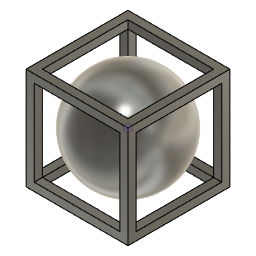
boxspherical (Autodesk Fusion 360 design; units mm, degrees)
Autodesk Fusion 360 part; units mm, degrees
sketch "Sketch1" plane through (0, 0, 0) normal (0, 1, 0) x (1, 0, 0)
  line L0 (12.5, -12.5) -> (-12.5, -12.5)
  line L1 (-12.5, -12.5) -> (-12.5, 12.5)
  line L2 (-12.5, 12.5) -> (12.5, 12.5)
  line L3 (12.5, 12.5) -> (12.5, -12.5)
  line L4 (12.5, -12.5) -> (-12.5, 12.5) construction
  line L5 (-12.5, -12.5) -> (12.5, 12.5) construction
  dimension "d1" = 25
  dimension "d2" = 25
  constraint horizontal L0
  constraint perpendicular L0 L1
  constraint parallel L0 L2
  constraint parallel L1 L3
  constraint coincident L4 origin
  constraint coincident L5 origin
  measures "d1" distance of L0.end L1.end
  measures "d2" distance of L1.end L2.end
extrude "Extrude1" add sketch "Sketch1" along normal mid plane 25 makes body 1
sketch "Sketch2" plane through (0, -12.5, 0) normal (0, -1, 0) x (1, 0, 0)
  line L0 (-12.5, -12.5) -> (12.5, -12.5)
  line L1 (12.5, -12.5) -> (12.5, 12.5)
  line L2 (12.5, 12.5) -> (-12.5, 12.5)
  line L3 (-12.5, 12.5) -> (-12.5, -12.5)
  line L4 (-10.5, -10.5) -> (10.5, -10.5)
  line L5 (10.5, -10.5) -> (10.5, 10.5)
  line L6 (10.5, 10.5) -> (-10.5, 10.5)
  line L7 (-10.5, 10.5) -> (-10.5, -10.5)
  dimension "d6" = -2
extrude "Extrude2" cut sketch "Sketch2" against normal blind 45 contours L4 L5 L6 L7 bodies 1
sketch "Sketch3" plane through (0, 0, 12.5) normal (0, 0, 1) x (-1, 0, 0)
  line L0 (12.5, 12.5) -> (-12.5, 12.5)
  line L1 (-12.5, 12.5) -> (-12.5, -12.5)
  line L2 (-12.5, -12.5) -> (12.5, -12.5)
  line L3 (12.5, -12.5) -> (12.5, 12.5)
  line L4 (10.5, 10.5) -> (-10.5, 10.5)
  line L5 (-10.5, 10.5) -> (-10.5, -10.5)
  line L6 (-10.5, -10.5) -> (10.5, -10.5)
  line L7 (10.5, -10.5) -> (10.5, 10.5)
  dimension "d9" = -2
extrude "Extrude3" cut sketch "Sketch3" against normal blind 41 contours L4 L5 L6 L7 bodies 1
sketch "Sketch4" plane through (12.5, 0, 0) normal (1, 0, 0) x (0, 1, 0)
  line L0 (-12.5, 12.5) -> (-12.5, -12.5)
  line L1 (-12.5, -12.5) -> (12.5, -12.5)
  line L2 (12.5, -12.5) -> (12.5, 12.5)
  line L3 (12.5, 12.5) -> (-12.5, 12.5)
  line L4 (-10.5, -10.5) -> (10.5, -10.5)
  line L5 (10.5, -10.5) -> (10.5, 10.5)
  line L6 (10.5, 10.5) -> (-10.5, 10.5)
  line L7 (-10.5, 10.5) -> (-10.5, -10.5)
  dimension "d12" = -2
extrude "Extrude4" cut sketch "Sketch4" against normal blind 38 contours L4 L5 L6 L7 bodies 1
sketch "Sketch5" plane through (0, 0, 0) normal (0, 1, 0) x (1, 0, 0)
sphere "SpherePrimitive1" add diameter 25 placed x (1, 0, 0) y (0, 0, -1) z (0, 1, 0) at (0, 0, 0) separate body makes body 2
equation "d3 = 25 mm / 2"
